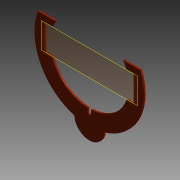
# Autodesk Inventor part: gyroYoke01
Saved by Autodesk Inventor 2013 (Build 170138000, 138)
## iProperties
Created: 2013-02-24
Part Number: gyroYoke01
Material: Wood (Oak)
Document SubType Name: Modeling
Designer: Nano
Density: 0.56 g/cm^3
Mass: 146.727 g
Surface Area: 937.732 cm^2
Volume: 262.012 cm^3
d0: 0.125 in
d1: 1.000 in
d3: 0.250 in
d4: 0.00 deg
d5: 0.250 in
d6: 0.250 in
d7: 0.250 in
d8: 0.250 in
Author: Nano
Autodesk Inventor part; units mm, degrees
ref_plane "YZ Plane" through (0, 0, 0) normal (1, 0, 0) x (0, 1, 0)
ref_plane "XZ Plane" through (0, 0, 0) normal (0, 1, 0) x (-1, 0, 0)
ref_plane "XY Plane" through (0, 0, 0) normal (0, 0, 1) x (1, 0, 0)
ref_plane "Work Plane1" through (0, 0, 0) normal (0, 0, 1) x (1, 0, 0)
sketch "Sketch1" plane through (0, 0, 0) normal (0, 0, 1) x (1, 0, 0)
  circle A0 centre (166.6875, 44.45) radius 6.35 construction
  line L0 (0, 0) -> (333.375, 0) construction
  line L1 (333.375, 0) -> (333.375, 88.9) construction
  line L2 (0, 88.9) -> (333.375, 88.9) construction
  line L3 (0, 0) -> (0, 88.9) construction
  line L4 (336.55, 95.25) -> (336.55, -6.35)
  line L5 (-3.175, -6.35) -> (-3.175, 95.25)
  arc A1 (361.952, -28.5758) -> (361.6406, 118.3031) centre (166.6875, 44.45) ccw
  arc A2 (109.447, -157.0949) -> (223.6431, -156.0919) centre (166.5241, -154.21) ccw
  arc A3 (223.6431, -156.0919) -> (361.952, -28.5758) centre (166.6875, 44.45) ccw
  arc A4 (-29.5537, -28.941) -> (109.447, -157.0949) centre (166.6875, 44.45) ccw
  arc A5 (-29.5402, 117.8769) -> (-29.5537, -28.941) centre (166.6875, 44.45) ccw
  arc A6 (336.55, 165.3087) -> (333.375, 169.6513) centre (166.6875, 44.45) ccw
  arc A7 (0, 169.6513) -> (-3.175, 165.3087) centre (166.6875, 44.45) ccw
  line L6 (361.6406, 118.3031) -> (296.5092, 118.3031)
  line L7 (35.5855, 117.8769) -> (-29.5402, 117.8769)
  arc A8 (194.8672, -103.8723) -> (308.8598, -6.35) centre (166.6875, 44.45) ccw
  arc A9 (307.1415, 95.25) -> (296.5092, 118.3031) centre (166.6875, 44.45) ccw
  arc A10 (35.5855, 117.8769) -> (25.271, 95.25) centre (166.6875, 44.45) ccw
  arc A11 (24.5152, -6.35) -> (136.5493, -103.4867) centre (166.6875, 44.45) ccw
  line L8 (-3.175, 95.25) -> (25.271, 95.25)
  line L9 (307.1415, 95.25) -> (336.55, 95.25)
  line L10 (336.55, -6.35) -> (308.8598, -6.35)
  line L11 (24.5152, -6.35) -> (-3.175, -6.35)
  line L12 (173.0375, -106.3919) -> (173.0375, -125.2673)
  line L13 (173.0375, -125.2673) -> (160.3375, -125.2673)
  line L14 (160.3375, -125.2673) -> (160.3375, -106.3919)
  line L15 (163.5125, -117.9837) -> (169.8625, -117.9837) projected
  line L16 (166.6875, 44.45) -> (38.9307, -83.3068) projected
  arc A12 (136.5493, -103.4867) -> (160.3375, -106.3919) centre (166.6875, 44.45) ccw
  arc A13 (173.0375, -106.3919) -> (194.8672, -103.8723) centre (166.6875, 44.45) ccw
  point P0 (166.6875, -117.9837)
  dimension "d0" = 3.175
  dimension "d5" = 6.35
  dimension "d6" = 6.35
  dimension "d7" = 6.35
  dimension "d8" = 6.35
  dimension "d9" = 3.175
  dimension "d10" = 3.175
  dimension "d11" = 6.35
  dimension "d12" = 6.35
  constraints: 26 point on circle, 22 end point, 13 centre point, 4 point on line, 1 coincident, 1 parallel, 1 other
  measures "d0" distance between parallel lines of L4 L1
  measures "d5" distance between parallel lines of L2 L9
  measures "d6" distance between parallel lines of L0 L10
  measures "d7" distance between parallel lines of L2 L8
  measures "d8" distance between parallel lines of L0 L11
  measures "d9" distance from line of L14 L15.start
  measures "d10" distance from line of L15.end L12
  measures "d11" distance from line of L12 point (166.688, -117.984)
  measures "d12" distance from line of point (166.688, -117.984) L14
extrude "Extrusion1" add sketch "Sketch1" against normal blind 6.35
sketch "Sketch2" plane through (0, 0, 0) normal (0, 0, 1) x (1, 0, 0)
  line L0 (339.725, 79.375) -> (346.075, 79.375)
  line L1 (346.075, 85.725) -> (346.075, 79.375)
  line L2 (346.075, 85.725) -> (339.725, 85.725)
  line L3 (339.725, 85.725) -> (339.725, 79.375)
  line L4 (339.725, 66.675) -> (346.075, 66.675)
  line L5 (346.075, 73.025) -> (346.075, 66.675)
  line L6 (346.075, 73.025) -> (339.725, 73.025)
  line L7 (339.725, 73.025) -> (339.725, 66.675)
  line L8 (339.725, 53.975) -> (346.075, 53.975)
  line L9 (346.075, 60.325) -> (346.075, 53.975)
  line L10 (346.075, 60.325) -> (339.725, 60.325)
  line L11 (339.725, 60.325) -> (339.725, 53.975)
  line L12 (346.075, 47.625) -> (339.725, 47.625)
  line L13 (339.725, 47.625) -> (339.725, 41.275)
  line L14 (339.725, 41.275) -> (346.075, 41.275)
  line L15 (346.075, 47.625) -> (346.075, 41.275)
  line L16 (346.075, 34.925) -> (339.725, 34.925)
  line L17 (339.725, 34.925) -> (339.725, 28.575)
  line L18 (339.725, 28.575) -> (346.075, 28.575)
  line L19 (346.075, 34.925) -> (346.075, 28.575)
  line L20 (346.075, 22.225) -> (339.725, 22.225)
  line L21 (339.725, 22.225) -> (339.725, 15.875)
  line L22 (339.725, 15.875) -> (346.075, 15.875)
  line L23 (346.075, 22.225) -> (346.075, 15.875)
  line L24 (346.075, 9.525) -> (339.725, 9.525)
  line L25 (339.725, 9.525) -> (339.725, 3.175)
  line L26 (339.725, 3.175) -> (346.075, 3.175)
  line L27 (346.075, 9.525) -> (346.075, 3.175)
  point P0 (0, 0)
extrude "Extrusion2" cut sketch "Sketch2" against normal blind 6.35
equation "\"d6\" = d5"
equation "\"d7\" = d5"
equation "\"d8\" = d5"
equation "\"d10\" = d9"
body "Solid1"
